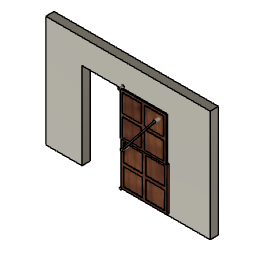
Evolution Door v9 (Autodesk Fusion 360 design; units mm, degrees)
Autodesk Fusion 360 part; units mm, degrees
sketch "main sketch" plane through (0, 0, 0) normal (0, 1, 0) x (1, 0, 0) in component "wall"
  line L0 (0, 0) -> (50, 0)
  line L1 (50, 0) -> (50, -50)
  line L2 (50, -50) -> (0, -50)
  line L3 (0, -50) -> (0, 0)
  line L4 (0, -50) -> (50, -50)
  line L5 (50, -50) -> (50, -100)
  line L6 (50, -100) -> (0, -100)
  line L7 (0, -100) -> (0, -50)
  line L8 (50, -100) -> (-30, -100)
  line L9 (-30, -100) -> (-30, -120)
  line L10 (-30, -120) -> (50, -120)
  line L11 (50, -120) -> (50, -100)
  line L12 (-30, -100) -> (0, -100)
  line L13 (0, -100) -> (0, 0)
  line L14 (0, 0) -> (-30, 0)
  line L15 (-30, 0) -> (-30, -100)
  line L16 (50, -120) -> (150, -120)
  line L17 (150, -120) -> (150, 0)
  line L18 (150, 0) -> (50, 0)
  line L19 (50, 0) -> (50, -120)
  line L20 (-30, -120) -> (150, -120)
  line L21 (150, -120) -> (150, -130)
  line L22 (150, -130) -> (-30, -130)
  line L23 (-30, -130) -> (-30, -120)
  line L24 (45, -95) -> (5, -95)
  line L25 (5, -95) -> (5, -55)
  line L26 (5, -55) -> (45, -55)
  line L27 (45, -55) -> (45, -95)
  line L28 (5, -5) -> (5, -45)
  line L29 (45, -5) -> (5, -5)
  line L30 (5, -45) -> (45, -45)
  line L31 (45, -45) -> (45, -5)
  line L32 (25, -95) -> (25, -21.7564)
  line L33 (25, -21.7564) -> (25, 0)
  line L34 (0, -75) -> (50, -75)
  line L35 (0, -25) -> (50, -25)
  line L36 (53, -47) -> (-3, -47)
  line L37 (-3, -47) -> (-3, -103)
  line L38 (-3, -103) -> (53, -103)
  line L39 (53, -103) -> (53, -47)
  line L40 (53, -47) -> (-3, -103) construction
  line L41 (-3, -47) -> (53, -103) construction
  line L42 (53, -53) -> (-3, -53)
  line L43 (-3, -53) -> (-3, 3)
  line L44 (-3, 3) -> (53, 3)
  line L45 (53, 3) -> (53, -53)
  line L46 (53, -53) -> (-3, 3) construction
  line L47 (-3, -53) -> (53, 3) construction
  circle A0 centre (-3, -103) radius 1.5
  line L48 (45, -95) -> (5, -45)
  line L49 (5, -55) -> (45, -5)
  circle A1 centre (45, -5) radius 1.5
  circle A2 centre (5, -45) radius 1.5
  circle A3 centre (5, -55) radius 1.5
  circle A4 centre (45, -95) radius 1.5
  line L50 (50, -50) -> (53.7444, -50)
  line L51 (0, -50) -> (-3, -50.0003)
  circle A5 centre (-3, 3) radius 1.5
  line L52 (5, -45) -> (5.4685, -45.5857)
  line L53 (45, -5) -> (46.0607, -6.0607)
  line L54 (5, -45) -> (6.0607, -46.0607)
  line L55 (5, -45) -> (6.5, -45) construction
  line L56 (5, -55) -> (6.0607, -56.0607)
  line L57 (5.5303, -55.5303) -> (45.5303, -5.5303)
  line L58 (5, -55) -> (3.9393, -53.9393)
  line L59 (4.4697, -54.4697) -> (44.4697, -4.4697)
  line L60 (45, -5) -> (43.8287, -4.063)
  line L61 (4.4697, -45.5303) -> (44.5662, -95.651)
  line L62 (45, -95) -> (46.0607, -93.9393)
  line L63 (5.6338, -44.599) -> (45.7303, -94.7197)
  line L64 (5.6338, -44.599) -> (5.526, -44.474)
  line L65 (44.5662, -95.651) -> (45.7303, -94.7197)
  line L66 (4.4697, -45.5303) -> (5.526, -44.474)
  line L67 (53, -103) -> (53, -134.5112)
  line L68 (-3, -103) -> (-3, -153.2356)
  line L69 (53, -130) -> (-97, -130)
  line L70 (-97, -130) -> (-97, 0)
  line L71 (-97, 0) -> (0, 0)
  line L72 (-30, -100) -> (-80, -100)
  line L73 (-80, -100) -> (-80, 0)
  line L74 (0, -100) -> (-50, -100)
  line L75 (-50, -100) -> (-48.5, -100)
  line L76 (-48.5, 0) -> (-50, 0)
  line L77 (-50, 0) -> (-50, -100)
  line L78 (53, -130) -> (103, -130)
  line L79 (103, -130) -> (103, 0)
  line L80 (-3, 3) -> (-3, 5.5)
  line L81 (-3, 5.5) -> (53, 5.5)
  line L82 (53, 3) -> (53, 5.5)
  line L83 (53, 5.5) -> (103, 5.5)
  line L84 (103, 5.5) -> (103, 0)
  line L85 (-3, 5.5) -> (-97, 5.5)
  line L86 (-97, 5.5) -> (-97, 0)
  line L87 (-4.7443, 5.5) -> (-4.7287, -130)
  line L88 (-50, 0) -> (-50, 5.5)
  point P0 (25, -75)
  point P1 (25, -25)
  dimension "d1" = 50
  dimension "d2" = 50
  dimension "d3" = 50
  dimension "d4" = 50
  dimension "d5" = 80
  dimension "d6" = 20
  dimension "d7" = 100
  dimension "d8" = 180
  dimension "d9" = 10
  dimension "d20" = 40
  dimension "d21" = 40
  dimension "d30" = 56
  dimension "d31" = 56
  dimension "d32" = 56
  dimension "d33" = 56
  dimension "d34" = 3
  dimension "d36" = 3
  dimension "d37" = 3
  dimension "d38" = 3
  dimension "d39" = 3
  dimension "d46" = 3
  dimension "d65" = 0.75
  dimension "d66" = 45
  dimension "d79" = 150
  dimension "d80" = 130
  dimension "d81" = 50
  dimension "d82" = 50
  dimension "d83" = 50
  dimension "d84" = 2.5
  constraint horizontal L0
  constraint vertical L1
  constraint horizontal L2
  constraint vertical L3
  constraint coincident L0.start L3.end
  constraint horizontal L4
  constraint vertical L5
  constraint horizontal L6
  constraint vertical L7
  constraint horizontal L8
  constraint vertical L9
  constraint horizontal L10
  constraint vertical L11
  constraint horizontal L12
  constraint vertical L13
  constraint horizontal L14
  constraint vertical L15
  constraint horizontal L16
  constraint vertical L17
  constraint horizontal L18
  constraint vertical L19
  constraint horizontal L20
  constraint vertical L21
  constraint horizontal L22
  constraint vertical L23
  constraint horizontal L24
  constraint perpendicular L24 L25
  constraint parallel L24 L26
  constraint parallel L25 L27
  constraint symmetric L4 L24.start L29.start
  constraint symmetric L4 L24.end L28.start
  constraint symmetric L4 L25.end L28.end
  constraint symmetric L4 L26.end L30.end
  constraint midpoint L24 L32.start
  constraint perpendicular L30 L32
  constraint midpoint L0 L33.end
  constraint perpendicular L0 L33
  constraint midpoint L7 L34.start
  constraint midpoint L5 L34.end
  constraint midpoint L3 L35.start
  constraint midpoint L1 L35.end
  constraint horizontal L36
  constraint perpendicular L36 L37
  constraint parallel L36 L38
  constraint parallel L37 L39
  constraint coincident L40 P0
  constraint coincident L41 P0
  constraint midpoint L34 P0
  constraint horizontal L42
  constraint perpendicular L42 L43
  constraint parallel L42 L44
  constraint parallel L43 L45
  constraint coincident L46 P1
  constraint coincident L47 P1
  constraint midpoint L35 P1
  constraint coincident L37.end L38.start
  constraint coincident L29.start L31.end
  constraint coincident L28.end L30.start
  constraint coincident L25.end L26.start
  constraint coincident L24.start L27.end
  constraint horizontal L50
  constraint coincident L43 L51.end
  constraint coincident L43.end L44.start
  constraint parallel L48 L52
  constraint coincident A1 L53.end
  constraint perpendicular L47 L53
  constraint horizontal L55
  constraint coincident A3 L56.end
  constraint coincident L41 L56.end
  constraint parallel L41 L56
  constraint midpoint L56 L57.start
  constraint midpoint L53 L57.end
  constraint coincident A3 L58.end
  constraint coincident L41 L58.end
  constraint midpoint L58 L59.start
  constraint parallel L57 L59
  constraint coincident A1 L60.end
  constraint perpendicular L59 L60
  constraint coincident L47 L61.start
  constraint parallel L48 L61
  constraint coincident A4 L62.end
  constraint perpendicular L41 L62
  constraint symmetric L48 L61.start L63.start
  constraint coincident L47 L64.end
  constraint perpendicular L63 L65
  constraint parallel L47 L66
  constraint perpendicular L22 L67
  constraint perpendicular L22 L68
  constraint coincident L22 L69.start
  constraint coincident L67 L69.start
  constraint perpendicular L23 L69
  constraint perpendicular L69 L70
  constraint perpendicular L9 L72
  constraint coincident L71 L73.end
  constraint perpendicular L71 L73
  constraint perpendicular L15 L74
  constraint horizontal L75
  constraint horizontal L76
  constraint vertical L77
  constraint midpoint L71 L76.start
  constraint perpendicular L67 L78
  constraint coincident L18 L79.end
  constraint perpendicular L18 L79
  constraint parallel L43 L80
  constraint perpendicular L45 L81
  constraint perpendicular L81 L82
  constraint perpendicular L79 L83
  constraint perpendicular L18 L84
  constraint perpendicular L70 L85
  constraint perpendicular L71 L86
  constraint coincident L85 L87.start
  constraint coincident L69 L87.end
  constraint midpoint L85 L88.end
  measures "d1" distance of L0.start L0.end
  measures "d2" distance of L0.start L2.end
  measures "d3" distance of L2.end L1.end
  measures "d4" distance of L2.end L6.end
  measures "d5" distance of L5.end L8.end
  measures "d6" distance of L5.end L10.end
  measures "d7" distance of L10.end L16.end
  measures "d8" distance of L9.end L16.end
  measures "d9" distance of L9.end L22.end
  measures "d20" distance of L25.end L26.end
  measures "d21" distance of L24.end L25.end
  measures "d30" distance of L37.end L38.end
  measures "d31" distance of L36.end L37.end
  measures "d32" distance of L43.end L44.end
  measures "d33" distance of L42.end L43.end
  measures "d34" diameter of A0
  measures "d36" diameter of A1
  measures "d37" diameter of A2
  measures "d38" diameter of A3
  measures "d39" diameter of A4
  measures "d46" diameter of A5
  measures "d65" distance of L28.end L52.end
  measures "d66" angle of L54 L55
  measures "d79" distance of L69.start L69.end
  measures "d80" distance of L69.end L70.end
  measures "d81" distance of L8.end L72.end
  measures "d82" distance of L6.end L74.end
  measures "d83" distance of L69.start L78.end
  measures "d84" distance of L43.end L80.end
extrude "Extrude1" add sketch "main sketch" along normal blind -4 and the other way blind 2 contours L0 L3 L13 L28 L29 L33 L35 | L0 L1 L19 L29 L31 L33 L35 A1 | L3 L13 L28 L35 L36 A2 L61 | L28 L29 L32 L33 L35 | L29 L32 L33 L35 A1 L59 | L2 L3 L4 L13 L36 L61 | L28 L30 L32 L35 A2 L59 | L1 L19 L30 L31 L32 L35 L36 | L29 A1 L59 L60 | L29 A1 L59 | L36 L48 A2 L61 | L36 L48 L59 L61 | L28 L30 A2 L63 L64 L66 | L28 A2 L61 L66 | L32 L35 L59 | L1 L2 L4 L19 L32 L36 | L31 L35 A1 L57 | L30 L31 L32 L35 L57 | L29 L59 L60 | L29 L49 A1 L59 | A1 L53 L60 | L35 L49 A1 L59 | L2 L4 L48 L59 | L36 L48 A2 L63 | L36 L48 L59 L63 | L48 A2 L52 L61 L66 | L30 L63 L64 L66 | L48 A2 L52 L54 | L30 A2 L54 L63 | L30 A2 L63 | L30 L36 A2 L59 L63 | L32 L35 L49 L59 | L30 L32 L49 L59 | L30 L32 L36 L57 | L2 L4 L32 L36 L57 | L31 A1 L57 | L31 A1 L53 L57 | L32 L35 L49 L57 | L35 L49 A1 L57 | L31 L53 L57 | L31 L49 A1 L57 | L2 L4 L49 L63 | L48 L49 L59 L63 | L36 L59 L63 | L30 L36 L49 L59 | L30 L32 L49 L57 | L30 L32 L57 | L36 L49 L57 L63 | L30 L36 L49 L57 | L36 L49 L59 L63 makes body 1 in component "bottom part"
extrude "Extrude1'" add sketch "main sketch" against normal blind 2 separate body contours L2 L4 L7 L13 L42 L59 | L42 L49 L59 L61 | L2 L4 L49 L61 | L7 L13 L25 L34 L42 A3 L59 | L2 L4 L5 L19 L32 L42 | L2 L4 L48 L57 | L48 L49 L57 L61 | L42 L49 A3 L59 | L42 L49 L57 L61 | L5 L6 L7 L8 L13 L19 L24 L25 L27 L34 A4 | L2 L4 L32 L42 L63 | L5 L19 L26 L27 L32 L34 L42 | L42 L48 L57 L63 | L42 L48 L57 L61 | L42 L49 A3 L57 | A3 L58 L59 | L49 A3 L58 L59 | L42 L57 L61 | L24 L25 L32 L34 | L25 L26 L32 L34 A3 L61 | L26 L32 L42 L63 | L26 L42 L48 L63 | L26 L42 L48 L61 | L26 L42 A3 L57 L61 | L26 L49 A3 L57 | L25 A3 L58 | L25 A3 L56 | L24 L32 L34 A4 L61 | L32 L34 L61 | L26 L32 L63 | L26 L27 L32 L34 L63 | L27 L34 A4 L63 | L26 L32 L48 L63 | L26 L32 L48 L61 | L26 A3 L57 | L26 L56 L57 | L26 A3 L56 L57 | L32 L34 L48 L61 | L34 L48 A4 L61 | L32 L34 L48 L63 | L27 A4 L62 L63 | L27 A4 L63 | L34 L48 A4 L63 | L24 A4 L61 | L24 A4 L61 L62 L63 L65 | L24 L48 A4 L61 | L27 L62 L63 | L27 L48 A4 L63 | L24 L61 L62 L63 L65 makes body 2 in component "upper part"
delete_body "RemoveBody1" bodies 2 in component "upper part"
delete_body "RemoveBody1'" bodies 1 in component "bottom part"
extrude "Extrude2" add sketch "main sketch" against normal blind 2 separate body contours L0 L14 L18 L43 L44 L45 A5 L71 | L0 L3 L13 L28 L29 L33 L35 | L3 L13 L14 L36 L43 L71 | L0 L1 L19 L29 L31 L33 L35 A1 | L3 L13 L28 L35 L36 A2 L61 | L1 L18 L19 L36 L45 | L28 L29 L32 L33 L35 | L29 L32 L33 L35 A1 L59 | L2 L3 L4 L13 L36 L61 | L3 L13 L36 L37 L43 L51 | L28 L30 L32 L35 A2 L59 | L1 L19 L30 L31 L32 L35 L36 | L29 A1 L59 L60 | L29 A1 L59 | L36 L48 A2 L61 | L36 L48 L59 L61 | L28 L30 A2 L63 L64 L66 | L28 A2 L61 L66 | L32 L35 L59 | L1 L19 L36 L39 L45 L50 | L1 L2 L4 L19 L32 L36 | L31 L35 A1 L57 | L30 L31 L32 L35 L57 | L29 L59 L60 | L29 L49 A1 L59 | A1 L53 L60 | L35 L49 A1 L59 | L2 L4 L48 L59 | L36 L48 A2 L63 | L36 L48 L59 L63 | L48 A2 L52 L61 L66 | L30 L63 L64 L66 | L48 A2 L52 L54 | L30 A2 L54 L63 | L30 A2 L63 | L30 L36 A2 L59 L63 | L32 L35 L49 L59 | L30 L32 L49 L59 | L30 L32 L36 L57 | L2 L4 L32 L36 L57 | L31 A1 L57 | L31 A1 L53 L57 | L32 L35 L49 L57 | L35 L49 A1 L57 | L31 L53 L57 | L31 L49 A1 L57 | L2 L4 L49 L63 | L48 L49 L59 L63 | L36 L59 L63 | L30 L36 L49 L59 | L30 L32 L49 L57 | L30 L32 L57 | L36 L49 L57 L63 | L30 L36 L49 L57 | L36 L49 L59 L63 makes body 3 in component "bottom part"
extrude "Extrude3" add sketch "main sketch" along normal blind -2 and the other way blind 4 separate body contours L2 L4 L7 L13 L42 L59 | L7 L13 L37 L42 L43 L51 | L42 L49 L59 L61 | L2 L4 L49 L61 | L7 L13 L25 L34 L42 A3 L59 | L7 L8 L12 L13 L37 L42 L74 | L6 L8 L11 L12 L19 L37 L38 A0 L74 | L2 L4 L5 L19 L32 L42 | L5 L19 L39 L42 L45 L50 | L2 L4 L48 L57 | L48 L49 L57 L61 | L42 L49 A3 L59 | L42 L49 L57 L61 | L5 L6 L7 L8 L13 L19 L24 L25 L27 L34 A4 | L37 L38 A0 | L37 A0 L68 | L2 L4 L32 L42 L63 | L5 L11 L19 L38 L39 L42 | L5 L19 L26 L27 L32 L34 L42 | L42 L48 L57 L63 | L42 L48 L57 L61 | L42 L49 A3 L57 | A3 L58 L59 | L49 A3 L58 L59 | L42 L57 L61 | L24 L25 L32 L34 | L25 L26 L32 L34 A3 L61 | L38 A0 L68 | L26 L32 L42 L63 | L26 L42 L48 L63 | L26 L42 L48 L61 | L26 L42 A3 L57 L61 | L26 L49 A3 L57 | L25 A3 L58 | L25 A3 L56 | L24 L32 L34 A4 L61 | L32 L34 L61 | L26 L32 L63 | L26 L27 L32 L34 L63 | L27 L34 A4 L63 | L26 L32 L48 L63 | L26 L32 L48 L61 | L26 A3 L57 | L26 L56 L57 | L26 A3 L56 L57 | L32 L34 L48 L61 | L34 L48 A4 L61 | L32 L34 L48 L63 | L27 A4 L62 L63 | L27 A4 L63 | L34 L48 A4 L63 | L24 A4 L61 | L24 A4 L61 L62 L63 L65 | L24 L48 A4 L61 | L27 L62 L63 | L27 L48 A4 L63 | L24 L61 L62 L63 L65 makes body 4 in component "bottom part"
delete_body "RemoveBody2" bodies 4 in component "bottom part"
extrude "Extrude4" add sketch "main sketch" against normal blind 2 contours L43 A5 L80 | L43 L44 A5 | L44 A5 L80 bodies 3 in component "bottom part"
extrude "Extrude2'" add sketch "main sketch" along normal blind -4 and the other way blind 2 separate body contours L7 L13 L25 L34 L42 A3 L59 | L7 L8 L12 L13 L37 L42 L74 | L6 L8 L11 L12 L19 L37 L38 A0 L74 | L42 L49 A3 L59 | L5 L6 L7 L8 L13 L19 L24 L25 L27 L34 A4 | L37 L38 A0 | L37 A0 L68 | L5 L11 L19 L38 L39 L42 | L5 L19 L26 L27 L32 L34 L42 | L42 L49 A3 L57 | A3 L58 L59 | L49 A3 L58 L59 | L24 L25 L32 L34 | L25 L26 L32 L34 A3 L61 | L38 A0 L68 | L26 L32 L42 L63 | L26 L42 L48 L63 | L26 L42 L48 L61 | L26 L42 A3 L57 L61 | L26 L49 A3 L57 | L25 A3 L58 | L25 A3 L56 | L24 L32 L34 A4 L61 | L32 L34 L61 | L26 L32 L63 | L26 L27 L32 L34 L63 | L27 L34 A4 L63 | L26 L32 L48 L63 | L26 L32 L48 L61 | L26 A3 L57 | L26 L56 L57 | L26 A3 L56 L57 | L32 L34 L48 L61 | L34 L48 A4 L61 | L32 L34 L48 L63 | L27 A4 L62 L63 | L27 A4 L63 | L34 L48 A4 L63 | L24 A4 L61 | L24 A4 L61 L62 L63 L65 | L24 L48 A4 L61 | L27 L62 L63 | L27 L48 A4 L63 | L24 L61 L62 L63 L65 makes body 5 in component "upper part"
extrude "Extrude3'" add sketch "main sketch" along normal blind -2 and the other way blind 4 contours L2 L4 L7 L13 L42 L59 | L7 L13 L37 L42 L43 L51 | L42 L49 L59 L61 | L2 L4 L49 L61 | L2 L4 L5 L19 L32 L42 | L5 L19 L39 L42 L45 L50 | L2 L4 L48 L57 | L48 L49 L57 L61 | L42 L49 L57 L61 | L2 L4 L32 L42 L63 | L42 L48 L57 L63 | L42 L48 L57 L61 | L42 L57 L61 bodies 5 in component "upper part"
extrude "Extrude5" add sketch "main sketch" against normal blind 2 contours L2 L4 L7 L13 L42 L59 | L7 L13 L37 L42 L43 L51 | L42 L49 L59 L61 | L2 L4 L49 L61 | L2 L4 L5 L19 L32 L42 | L5 L19 L39 L42 L45 L50 | L2 L4 L48 L57 | L48 L49 L57 L61 | L42 L49 L57 L61 | L2 L4 L32 L42 L63 | L42 L48 L57 L63 | L42 L48 L57 L61 | L42 L57 L61 bodies 3 in component "bottom part"
extrude "Extrude4'" add sketch "main sketch" along normal blind -4.5 and the other way blind 2.3 contours L37 L38 A0 | L37 A0 L68 | L38 A0 L68 bodies 5 in component "upper part"
extrude "Extrude6" add sketch "main sketch" against normal blind 2.3 contours L43 A5 L80 | L43 L44 A5 | L44 A5 L80 bodies 3 in component "bottom part"
extrude "Extrude1''" add sketch "main sketch" against normal blind 7 separate body contours L29 A1 L59 L60 | L29 A1 L59 | L29 L59 L60 | L29 L49 A1 L59 | A1 L53 L60 | L31 A1 L57 | L31 A1 L53 L57 | L31 L53 L57 | L31 L49 A1 L57 | A3 L58 L59 | L49 A3 L58 L59 | L26 L49 A3 L57 | L25 A3 L58 | L25 A3 L56 | L26 A3 L57 | L26 L56 L57 | L26 A3 L56 L57 makes body 6 at (3.7201, -4.6667, 55.7822) makes body 7 at (46.4925, -2.3333, 4.8506) in component "bottom connecting bar"
extrude "Extrude2''" add sketch "main sketch" along normal blind -7 and the other way blind 5 contours L29 L59 L60 | L29 L49 A1 L59 | L35 L49 A1 L59 | L2 L4 L48 L59 | L42 L49 L59 L61 | L2 L4 L49 L61 | L32 L35 L49 L59 | L30 L32 L49 L59 | L32 L35 L49 L57 | L35 L49 A1 L57 | L31 L53 L57 | L31 L49 A1 L57 | L2 L4 L49 L63 | L2 L4 L48 L57 | L48 L49 L57 L61 | L48 L49 L59 L63 | L42 L49 A3 L59 | L42 L49 L57 L61 | L30 L36 L49 L59 | L30 L32 L49 L57 | L36 L49 L57 L63 | L30 L36 L49 L57 | L36 L49 L59 L63 | L42 L49 A3 L57 | L49 A3 L58 L59 | L26 L49 A3 L57 | L26 L56 L57 bodies 6 7 in component "bottom connecting bar"
extrude "Extrude1'''" add sketch "main sketch" against normal blind 10 separate body contours L28 L30 A2 L63 L64 L66 | L28 A2 L61 L66 | L48 A2 L52 L61 L66 | L30 L63 L64 L66 | L48 A2 L52 L54 | L30 A2 L54 L63 | L30 A2 L63 | L27 A4 L62 L63 | L27 A4 L63 | L24 A4 L61 | L24 A4 L61 L62 L63 L65 | L24 L48 A4 L61 | L27 L62 L63 | L27 L48 A4 L63 | L24 L61 L62 L63 L65 makes body 8 at (46.4095, -6.6667, 94.487) makes body 9 at (3.6178, -3.3333, 44.4173) in component "connecting bar"
extrude "Extrude2'''" add sketch "main sketch" along normal blind -10 and the other way blind 8 contours L36 L48 A2 L61 | L36 L48 L59 L61 | L2 L4 L48 L59 | L2 L4 L49 L61 | L36 L48 A2 L63 | L36 L48 L59 L63 | L48 A2 L52 L61 L66 | L30 L63 L64 L66 | L48 A2 L52 L54 | L30 A2 L54 L63 | L2 L4 L49 L63 | L2 L4 L48 L57 | L48 L49 L57 L61 | L48 L49 L59 L63 | L42 L48 L57 L63 | L42 L48 L57 L61 | L26 L42 L48 L63 | L26 L42 L48 L61 | L26 L32 L48 L63 | L26 L32 L48 L61 | L32 L34 L48 L61 | L34 L48 A4 L61 | L32 L34 L48 L63 | L34 L48 A4 L63 | L24 L48 A4 L61 | L27 L62 L63 | L27 L48 A4 L63 | L24 L61 L62 L63 L65 bodies 8 9 in component "connecting bar"
extrude "Extrude2''''" add sketch "main sketch" along normal blind 10 separate body contours L0 L14 L18 L43 L44 L45 A5 L71 | L0 L3 L13 L28 L29 L33 L35 | L3 L13 L14 L36 L43 L71 | L0 L1 L19 L29 L31 L33 L35 A1 | L3 L13 L28 L35 L36 A2 L61 | L8 L12 L14 L37 L43 L71 L74 L87 | L14 L43 A5 L71 L80 L85 L87 | L1 L18 L19 L36 L45 | L28 L29 L32 L33 L35 | L29 L32 L33 L35 A1 L59 | L2 L3 L4 L13 L36 L61 | L3 L13 L36 L37 L43 L51 | L28 L30 L32 L35 A2 L59 | L43 A5 L80 | L43 L44 A5 | L1 L19 L30 L31 L32 L35 L36 | L18 L45 L82 L83 L84 | L16 L18 L20 L39 L45 L67 L79 | L29 A1 L59 L60 | L29 A1 L59 | L2 L4 L7 L13 L42 L59 | L7 L13 L37 L42 L43 L51 | L36 L48 A2 L61 | L36 L48 L59 L61 | L28 L30 A2 L63 L64 L66 | L28 A2 L61 L66 | L32 L35 L59 | L8 L10 L12 L20 L37 A0 L68 L74 L87 | L44 A5 L80 | L44 A5 L80 L81 L82 | L1 L19 L36 L39 L45 L50 | L1 L2 L4 L19 L32 L36 | L31 L35 A1 L57 | L30 L31 L32 L35 L57 | L29 L59 L60 | L29 L49 A1 L59 | A1 L53 L60 | L35 L49 A1 L59 | L2 L4 L48 L59 | L42 L49 L59 L61 | L2 L4 L49 L61 | L7 L13 L25 L34 L42 A3 L59 | L7 L8 L12 L13 L37 L42 L74 | L36 L48 A2 L63 | L36 L48 L59 L63 | L48 A2 L52 L61 L66 | L30 L63 L64 L66 | L48 A2 L52 L54 | L30 A2 L54 L63 | L30 A2 L63 | L30 L36 A2 L59 L63 | L32 L35 L49 L59 | L30 L32 L49 L59 | L6 L8 L11 L12 L19 L37 L38 A0 L74 | L10 L20 L22 L68 L69 L87 | L2 L4 L5 L19 L32 L42 | L5 L19 L39 L42 L45 L50 | L30 L32 L36 L57 | L2 L4 L32 L36 L57 | L31 A1 L57 | L31 A1 L53 L57 | L32 L35 L49 L57 | L35 L49 A1 L57 | L16 L20 L22 L67 L78 L79 | L31 L53 L57 | L31 L49 A1 L57 | L2 L4 L49 L63 | L2 L4 L48 L57 | L48 L49 L57 L61 | L48 L49 L59 L63 | L42 L49 A3 L59 | L42 L49 L57 L61 | L5 L6 L7 L8 L13 L19 L24 L25 L27 L34 A4 | L36 L59 L63 | L30 L36 L49 L59 | L30 L32 L49 L57 | L37 L38 A0 | L37 A0 L68 | L10 L11 L19 L20 L38 A0 L68 | L10 L16 L20 L22 L67 L68 L69 | L2 L4 L32 L42 L63 | L5 L11 L19 L38 L39 L42 | L5 L19 L26 L27 L32 L34 L42 | L30 L32 L57 | L36 L49 L57 L63 | L30 L36 L49 L57 | L11 L16 L19 L20 L38 L67 | L42 L48 L57 L63 | L42 L48 L57 L61 | L36 L49 L59 L63 | L42 L49 A3 L57 | A3 L58 L59 | L49 A3 L58 L59 | L42 L57 L61 | L24 L25 L32 L34 | L25 L26 L32 L34 A3 L61 | L38 A0 L68 | L26 L32 L42 L63 | L26 L42 L48 L63 | L26 L42 L48 L61 | L26 L42 A3 L57 L61 | L26 L49 A3 L57 | L25 A3 L58 | L25 A3 L56 | L24 L32 L34 A4 L61 | L32 L34 L61 | L26 L32 L63 | L26 L27 L32 L34 L63 | L27 L34 A4 L63 | L26 L32 L48 L63 | L26 L32 L48 L61 | L26 A3 L57 | L26 L56 L57 | L26 A3 L56 L57 | L32 L34 L48 L61 | L34 L48 A4 L61 | L32 L34 L48 L63 | L27 A4 L62 L63 | L27 A4 L63 | L34 L48 A4 L63 | L24 A4 L61 | L24 A4 L61 L62 L63 L65 | L24 L48 A4 L61 | L27 L62 L63 | L27 L48 A4 L63 | L24 L61 L62 L63 L65 makes body 10 in component "wall"
extrude "Extrude3''" add sketch "main sketch" along normal blind 10 contours L8 L9 L10 L12 L20 L74 L87 | L9 L23 L69 L70 L71 L72 L73 L74 L75 | L71 L85 L86 L88 | L10 L20 L22 L23 L69 L87 | L71 L72 L73 L77 bodies 10 in component "wall"
extrude "Extrude5'" add sketch "main sketch" against normal blind 5 contours L37 L38 A0 | L37 A0 L68 | L38 A0 L68 sketch seen with x (1, 0, 0) y (0, 1, 0) z (0, 0, 1) at (0.0245, 0.0001, 0.0473) bodies 5 in component "upper part"
extrude "Extrude6'" cut 1 faces at (-3.2229, -4.9999, 103.9417) along direction (0, 1, 0) blind 5 on bodies 5 bodies 5 in component "upper part"
delete_face "DeleteFace1" 1 faces at (-1.7276, -3.5, 102.215) on bodies 5 in component "upper part"
extrude "Extrude7" cut 1 faces at (-3.21, -4.5, 103.8298) along direction (0, 1, 0) blind 3 on bodies 5 bodies 5 in component "upper part"
extrude "Extrude7'" cut 1 faces at (-2.584, -2.3, -3.1231) along direction (0, 1, 0) blind 2.3 on bodies 3 bodies 3 in component "bottom part"
move_face "OffsetFaces1" offset -2 1 faces at (44.6335, 0, 95.6348) on bodies 8 in component "connecting bar"
move_face "OffsetFaces1'" offset -2 1 faces at (4.2215, 0, 55.2817) on bodies 6 in component "bottom connecting bar"
extrude "Extrude4''" add sketch "main sketch" against normal blind 3 contours L43 A5 L80 | L43 L44 A5 | L44 A5 L80 | L37 L38 A0 | L37 A0 L68 | L38 A0 L68 bodies 10 in component "wall"
extrude "Extrude5''" add 1 faces at (-3.21, -3, 103.8298) along direction (0, -1, 0) blind 2 on bodies 10 bodies 10 in component "wall"
move_face "OffsetFaces1''" offset -3 1 faces at (34.3333, -0.6667, 53) on bodies 3 in component "bottom part"
sketch "upper part model" plane through (0, -4, 0) normal (0, -1, 0) x (1, 0, 0) in component "upper part"
  line L0 (53, 103) -> (-1.5, 103)
  arc A0 (-3, 101.5) -> (-1.5, 103) centre (-3, 103) ccw
  line L1 (-3, 101.5) -> (-3, 50.0003)
  line L2 (-3, 50.0003) -> (0, 50)
  line L3 (0, 50) -> (53, 50)
  line L4 (53, 50) -> (53, 103)
  line L5 (53, 103) -> (-3, 50.0003)
  line L6 (50, 100.0002) -> (0, 100.0002)
  line L7 (0, 100.0002) -> (0, 53.0002)
  line L8 (0, 53.0002) -> (50, 53.0002)
  line L9 (50, 53.0002) -> (50, 100.0002)
  line L10 (50, 100.0002) -> (0, 53.0002) construction
  line L11 (0, 100.0002) -> (50, 53.0002) construction
  line L12 (50, 78.5002) -> (0, 78.5002)
  line L13 (0, 78.5002) -> (0, 74.5002)
  line L14 (0, 74.5002) -> (50, 74.5002)
  line L15 (50, 74.5002) -> (50, 78.5002)
  line L16 (50, 78.5002) -> (0, 74.5002) construction
  line L17 (0, 78.5002) -> (50, 74.5002) construction
  line L18 (27, 100.0002) -> (23, 100.0002)
  line L19 (23, 100.0002) -> (23, 53.0002)
  line L20 (23, 53.0002) -> (27, 53.0002)
  line L21 (27, 53.0002) -> (27, 100.0002)
  line L22 (27, 100.0002) -> (23, 53.0002) construction
  line L23 (23, 100.0002) -> (27, 53.0002) construction
  point P0 (25, 76.5002)
  point P1 (25, 76.5002)
  point P2 (25, 76.5002)
  dimension "d146" = 50
  dimension "d147" = 47
  dimension "d148" = 4
  dimension "d149" = 4
  constraint coincident L0.start L4.end
  constraint coincident L1.end L2.start
  constraint horizontal L6
  constraint perpendicular L6 L7
  constraint parallel L6 L8
  constraint parallel L7 L9
  constraint coincident L10 P2
  constraint coincident L11 P2
  constraint midpoint L5 P2
  constraint horizontal L12
  constraint perpendicular L12 L13
  constraint parallel L12 L14
  constraint parallel L13 L15
  constraint coincident L16 P2
  constraint coincident L17 P2
  constraint coincident P2 P1
  constraint horizontal L18
  constraint perpendicular L18 L19
  constraint parallel L18 L20
  constraint parallel L19 L21
  constraint coincident L22 P2
  constraint coincident L23 P2
  measures "d146" distance of L7.end L8.end
  measures "d147" distance of L6.end L7.end
  measures "d148" distance of L12.end L13.end
  measures "d149" distance of L19.end L20.end
extrude "Extrude6''" cut sketch "upper part model" against normal blind 0.5 contours L0 A0 L1 L5 L6 L7 L8 L13 L18 | L2 L3 L4 L5 L6 L8 L9 L15 L20 | L5 L9 L12 L14 L15 L21 | L6 L12 L18 L19 L21 | L5 L14 L19 L21 | L5 L12 L19 L21 | L5 L7 L12 L13 L14 L19 | L8 L14 L19 L20 L21 sketch seen with x (1, 0, 0.000972) y (0, 1, 0) z (-0.000972, 0, 1) at (0.0757, -0.0001, -0.0443) bodies 10 in component "wall"
extrude "Extrude8" cut sketch "upper part model" against normal blind 0.5 contours L0 A0 L1 L5 L6 L7 L8 L13 L18 | L2 L3 L4 L5 L6 L8 L9 L15 L20 | L5 L9 L12 L14 L15 L21 | L6 L12 L18 L19 L21 | L5 L14 L19 L21 | L5 L12 L19 L21 | L5 L7 L12 L13 L14 L19 | L8 L14 L19 L20 L21 bodies 5 in component "upper part"
sketch "bottom part model" plane through (0, -2, 0) normal (0, -1, 0) x (1, 0, 0) in component "bottom part"
  arc A0 (-1.5, -3) -> (-3, -1.5) centre (-3, -3) ccw
  line L0 (-1.5, -3) -> (53, -3)
  line L1 (53, -3) -> (53, 50)
  line L2 (53, 50) -> (-3, 50)
  line L3 (-3, 50) -> (-3, -1.5)
  line L4 (-3, 50) -> (53, -3)
  line L5 (50, 47) -> (0, 47)
  line L6 (0, 47) -> (0, 0)
  line L7 (0, 0) -> (50, 0)
  line L8 (50, 0) -> (50, 47)
  line L9 (0, 47) -> (50, 0) construction
  line L10 (27, 47) -> (23, 47)
  line L11 (23, 47) -> (23, 0)
  line L12 (23, 0) -> (27, 0)
  line L13 (27, 0) -> (27, 47)
  line L14 (27, 47) -> (23, 0) construction
  line L15 (50, 25.5) -> (0, 25.5)
  line L16 (0, 25.5) -> (0, 21.5)
  line L17 (0, 21.5) -> (50, 21.5)
  line L18 (50, 21.5) -> (50, 25.5)
  line L19 (50, 25.5) -> (0, 21.5) construction
  point P0 (25, 23.5)
  point P1 (25, 23.5)
  point P2 (25, 23.5)
  dimension "d154" = 50
  dimension "d155" = 47
  dimension "d156" = 4
  dimension "d157" = 4
  constraint coincident L2.end L3.start
  constraint coincident L0.end L1.start
  constraint horizontal L5
  constraint perpendicular L5 L6
  constraint parallel L5 L7
  constraint parallel L6 L8
  constraint coincident L9 P2
  constraint midpoint L4 P2
  constraint horizontal L10
  constraint perpendicular L10 L11
  constraint parallel L10 L12
  constraint parallel L11 L13
  constraint coincident L14 P2
  constraint coincident P2 P1
  constraint horizontal L15
  constraint perpendicular L15 L16
  constraint parallel L15 L17
  constraint parallel L16 L18
  constraint coincident L19 P2
  measures "d154" distance of L6.end L7.end
  measures "d155" distance of L5.end L6.end
  measures "d156" distance of L11.end L12.end
  measures "d157" distance of L15.end L16.end
extrude "Extrude8'" add sketch "bottom part model" along normal blind 0.5 contours A0 L0 L3 L4 L5 L6 L7 L12 L16 | L1 L2 L4 L5 L7 L8 L10 L18 | L4 L8 L13 L15 L17 L18 | L7 L11 L12 L13 L17 | L4 L6 L11 L15 L16 L17 | L5 L10 L11 L13 L15 | L4 L11 L13 L17 | L4 L11 L13 L15 bodies 3 in component "bottom part"
move_face "OffsetFaces1'''" offset -3 1 faces at (-50, 3.3333, 29.6667) on bodies 10 in component "wall"
extrude "Extrude1''''" [suppressed] in component "wall"
extrude "Extrude1'''''" [suppressed] in component "door up"
extrude "Extrude1''''''" [suppressed] in component "door down"
component "wall" placed x (1, 0, 0) y (0, 1, 0) z (0, 0, 1) at (0.0245, 0.0001, 0.0473)
component "door" placed x (1, 0, 0) y (0, 1, 0) z (0, 0, 1) at (0, 0, 0)
component "connecting bar" placed x (0.999999, 0, 0.001517) y (0, 1, 0) z (-0.001517, 0, 0.999999) at (0.1519, 0, -0.0215)
component "upper part" placed x (1, 0, 0.000972) y (0, 1, 0) z (-0.000972, 0, 1) at (0.1001, 0, 0.0029) in component "door"
component "bottom part" placed x (0.999998, 0, -0.001745) y (0, 1, 0) z (0.001745, 0, 0.999998) at (0.0051, 0, -0.0052) in component "door"
named bodies: "door upper part", "bottom part", "upper part", "bottom bar", "upper bar", "wall"
